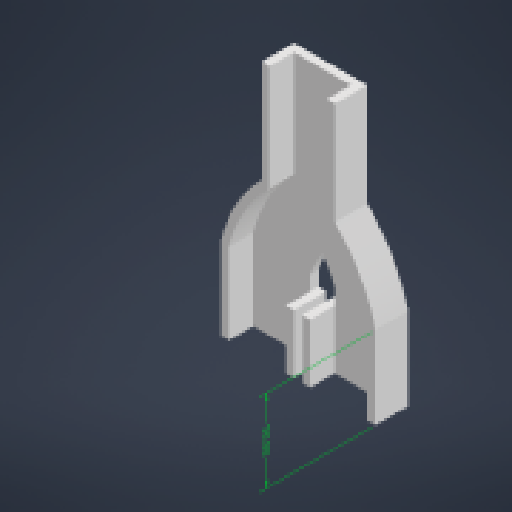
# Autodesk Inventor part: newmiddle
Saved by Autodesk Inventor 2026.2 (Build 302298000, 298)
## iProperties
Created: 2026-04-08
Part Number: newmiddle
Material: Generic
Document SubType Name: Modeling
Designer: danda
Density: 1 g/cm^3
Appearance: Default
Author: danda
Autodesk Inventor part; units mm, degrees
ref_plane "YZ Plane" through (0, 0, 0) normal (1, 0, 0) x (0, 1, 0)
ref_plane "XZ Plane" through (0, 0, 0) normal (0, 1, 0) x (-1, 0, 0)
ref_plane "XY Plane" through (0, 0, 0) normal (0, 0, 1) x (1, 0, 0)
sketch "Sketch1" plane through (0, 0, 0) normal (0, 0, 1) x (1, 0, 0)
  line L0 (46.2872, 31.5555) -> (46.2872, -28.4445)
  line L1 (11.2872, 31.5555) -> (11.2872, -28.4445)
  arc A0 (11.2872, -28.4445) -> (-13.7128, -71.7458) centre (73.6621, -93.3242) ccw
  line L2 (11.2872, -28.4445) -> (-13.7128, -71.7458) construction
  line L3 (11.2872, -28.4445) -> (61.2872, -28.4445) construction
  line L4 (-13.7128, -71.7458) -> (-13.7128, -121.7458)
  arc A1 (71.2872, -71.7458) -> (46.2872, -28.4445) centre (-16.0876, -93.3242) ccw
  line L5 (71.2872, -71.7458) -> (71.2872, -121.7458)
  line L6 (21.2872, -121.7458) -> (21.2872, -76.5352)
  arc A2 (28.7872, -61.5241) -> (21.2872, -76.5352) centre (73.6621, -93.3242) ccw
  arc A3 (36.2872, -76.5352) -> (28.7872, -61.5241) centre (-16.0876, -93.3242) ccw
  line L7 (36.2872, -76.5352) -> (36.2872, -121.7458)
  line L8 (-18.7128, -121.7458) -> (-18.7128, -71.1458)
  arc A4 (6.2872, -26.3494) -> (-18.7128, -71.1458) centre (73.6621, -93.3242) ccw
  line L9 (6.2872, -26.3494) -> (6.2872, 36.5555)
  line L10 (6.2872, 36.5555) -> (51.2872, 36.5555)
  line L11 (51.2872, 36.5555) -> (51.2872, -26.3494)
  arc A5 (76.2872, -71.1458) -> (51.2872, -26.3494) centre (-16.0876, -93.3242) ccw
  line L12 (76.2872, -71.1458) -> (76.2872, -121.7458)
  line L13 (-18.7128, -121.7458) -> (76.2872, -121.7458)
  line L14 (11.2872, 31.5555) -> (11.2872, 36.5555)
  line L15 (46.2872, 31.5555) -> (46.2872, 36.5555)
  line L16 (31.2872, -121.7458) -> (31.2872, -85.5895)
  line L17 (26.2872, -85.5895) -> (26.2872, -121.7458)
  line L18 (21.2872, -85.5895) -> (26.2872, -85.5895)
  line L19 (31.2872, -85.5895) -> (36.2872, -85.5895)
  line L20 (45.9283, 31.5555) -> (46.2872, 31.5555)
  point P0 (0, 0)
  dimension "d0" = 35
  dimension "d1" = 60
  dimension "d2" = 50
  dimension "d3" = 120
  dimension "d4" = 90
  dimension "d5" = 50
  dimension "d6" = 35
  dimension "d7" = 5
  dimension "d12" = 5
  constraints: 42 end point, 12 point on circle, 7 point on line, 6 centre point, 5 perpendicular, 3 horizontal, 2 vertical, 1 equal length, 7 other
  measures "d0" distance of L1.start L0.start
  measures "d1" distance of L0.start L0.end
  measures "d2" distance of L1.end L2.end
  measures "d3" angle of L2 L3
  measures "d4" radius of A0
  measures "d5" distance of L2.end L4.end
  measures "d6" distance between parallel lines of L4 L6
  measures "d7" distance between parallel lines of L1 L9
  measures "d12" distance between parallel lines of L7 L16
extrude "Extrusion1" add sketch "Sketch1" along normal blind 5 contours L0 A1 L5 L13 L7 A3 A2 L6 L4 A0 L1 L14 L10 L15
extrude "Extrusion2" add sketch "Sketch1" along normal blind 20 contours L15 L10 L11 A5 L12 L13 L5 A1 L0 | L14 L1 A0 L4 L13 L8 A4 L9 L10 | L13 L16 L19 L7 | L13 L6 L18 L17
body "Solid1"
